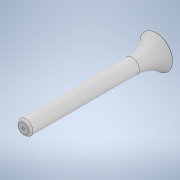
# Autodesk Inventor part: fiberHolder2
Saved by Autodesk Inventor 2022.2 (Build 262287000, 287)
## iProperties
Created: 2021-12-20
Part Number: fiberHolder2
Material: Generic
Document SubType Name: Modeling
Designer: Andrei
Density: 1 g/cm^3
Appearance: Default
Author: Andrei
Autodesk Inventor part; units mm, degrees
ref_plane "YZ Plane" through (0, 0, 0) normal (1, 0, 0) x (0, 1, 0)
ref_plane "XZ Plane" through (0, 0, 0) normal (0, 1, 0) x (-1, 0, 0)
ref_plane "XY Plane" through (0, 0, 0) normal (0, 0, 1) x (1, 0, 0)
sketch "Sketch1" plane through (0, 0, 0) normal (1, 0, 0) x (0, 1, 0)
  line L0 (10, 0) -> (10, 150)
  arc A0 (10, 0) -> (24.6447, -35.3553) centre (60, 0) ccw
  line L1 (10, 0) -> (60, 0) construction
  line L2 (24.6447, -35.3553) -> (60, 0) construction
  line L3 (24.6447, -35.3553) -> (0, -35.3553)
  line L4 (10, 150) -> (0, 150)
  line L5 (0, 150) -> (0, -35.3553)
  point P0 (0, 0)
  dimension "d5" = 50
  dimension "d6" = 45
  constraints: 12 end point, 2 point on circle, 1 centre point, 1 horizontal, 1 tangent, 1 vertical
  measures "d5" radius of A0
  measures "d6" angle of L1 L2
revolve "Revolution1" add sketch "Sketch1" angle 360 about axis through (0, 0, 150) along (0, 0, -1)
fillet "Fillet1" radius 3 1 edges at (0, -10, 150)
sketch "Sketch2" plane through (0, 0, 150) normal (0, 0, 1) x (1, 0, 0)
  point P0 (0, 0)
  point P1 (0, 0)
  constraints: 1 coincident
hole "Hole1" at (0, 0, 150) direction (0, 0, -1) diameter 3 end through all
fillet "Fillet2" radius 50 1 edges at (0, 1.5, -35.3553)
chamfer "Chamfer1" distance 3 angle 45 2 edges at (-24.6447, 0, -35.3553) (24.6447, 0, -35.3553)
equation "\"d5\" = Rbend"
equation "\"channelDiameter\" = 1"
equation "\"Rbend\" = 50"
body "Solid1"
